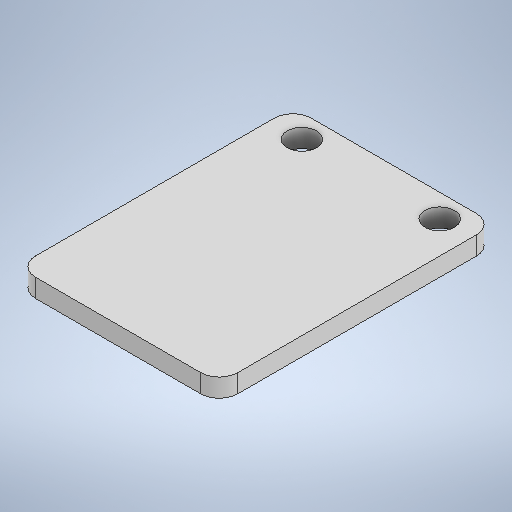
# Autodesk Inventor part: DFR0440
Saved by Autodesk Inventor 2025 (Build 290162010, 162A)
## iProperties
Created: 2025-02-16
Part Number: DFR0440
Material: Générique
Document SubType Name: Modeling
Designer: arthu
Density: 1 g/cm^3
Appearance: Par défaut
Author: arthu
Autodesk Inventor part; units mm, degrees
ref_plane "YZ Plane" through (0, 0, 0) normal (1, 0, 0) x (0, 1, 0)
ref_plane "XZ Plane" through (0, 0, 0) normal (0, 1, 0) x (-1, 0, 0)
ref_plane "XY Plane" through (0, 0, 0) normal (0, 0, 1) x (1, 0, 0)
sketch "Esquisse1" plane through (0, 0, 0) normal (0, 1, 0) x (-1, 0, 0)
  line L0 (0, 0) -> (22, 0)
  line L1 (22, 0) -> (22, -30)
  line L2 (22, -30) -> (0, -30)
  line L3 (0, -30) -> (0, 0)
  dimension "d0" = 22
  dimension "d1" = 30
  constraints: 8 end point, 2 parallel, 1 horizontal, 1 perpendicular
  measures "d0" distance of L1.end L2.end
  measures "d1" distance of L0.end L1.end
extrude "Extrusion1" add sketch "Esquisse1" along normal blind 2
sketch "Esquisse2" plane through (0, 2, 0) normal (0, 1, 0) x (1, 0, 0)
  line L0 (0, 30) -> (-22, 30) projected
  line L1 (-11, 30) -> (-3.5, 30)
  line L2 (-11, 30) -> (-18.5, 30)
  line L3 (-18.5, 30) -> (-18.5, 27.5)
  line L4 (-3.5, 30) -> (-3.5, 27.5)
  circle A0 centre (-18.5, 27.5) radius 1.6
  circle A1 centre (-3.5, 27.5) radius 1.6
  point P0 (0, 0)
  dimension "d4" = 7.5
  dimension "d5" = 7.5
  dimension "d6" = 2.5
  dimension "d7" = 2.5
  dimension "d8" = 3.2
  dimension "d9" = 3.2
  constraints: 8 end point, 2 centre point, 2 coincident, 2 point on line, 2 vertical, 1 midpoint
  measures "d4" distance of L1.start L1.end
  measures "d5" distance of L1.start L2.end
  measures "d6" distance of L2.end L3.end
  measures "d7" distance of L1.end L4.end
  measures "d8" diameter of A0
  measures "d9" diameter of A1
extrude "Extrusion2" cut sketch "Esquisse2" against normal through all
fillet "Congé1" radius 2 4 edges at (0, 1, -30) (-22, 1, -30) (0, 1, 0) (-22, 1, 0)
